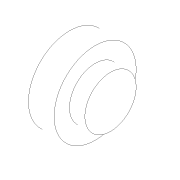
# Autodesk Inventor part: Remskive
Saved by Autodesk Inventor 2021 (Build 250183000, 183)
## iProperties
Created: 2020-11-11
Part Number: Remskive
Material: Steel
Document SubType Name: Modeling
Designer: Alfred Brauner
Density: 7.85 g/cm^3
Appearance: Plate
Mass: 87.7949 g
Surface Area: 32.4212 cm^2
Volume: 11.1841 cm^3
Author: Alfred Brauner
Autodesk Inventor part; units mm, degrees
ref_plane "YZ Plane" through (0, 0, 0) normal (1, 0, 0) x (0, 1, 0)
ref_plane "XZ Plane" through (0, 0, 0) normal (0, 1, 0) x (-1, 0, 0)
ref_plane "XY Plane" through (0, 0, 0) normal (0, 0, 1) x (1, 0, 0)
sketch "Sketch1" plane through (0, 0, 0) normal (0, 0, 1) x (1, 0, 0)
  line L0 (0, 0) -> (16, 0)
  line L1 (16, 0) -> (16, 10)
  line L2 (16, 10) -> (10, 10)
  line L3 (0, 0) -> (0, 16)
  line L4 (0, 16) -> (10, 16)
  line L5 (10, 16) -> (10, 10)
  dimension "d1" = 10
  dimension "d2" = 6
  dimension "d3" = 16
  dimension "d5" = 10
  constraints: 12 end point, 3 perpendicular, 2 horizontal, 1 vertical
  measures "d1" distance of L0.end L1.end
  measures "d2" distance of L1.end L2.end
  measures "d3" distance of L0.start L3.end
  measures "d5" distance between parallel lines of L3 L5
revolve "Revolution1" add sketch "Sketch1" angle 360 about axis through (0, 0, 0) along (1, 0, 0)
body "Solid1"
